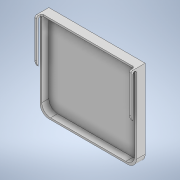
# Autodesk Inventor part: backpack
Saved by Autodesk Inventor 2021 (Build 250183000, 183)
## iProperties
Created: 2021-02-06
Part Number: backpack
Material: Generic
Document SubType Name: Modeling
Designer: allen
Density: 1 g/cm^3
Appearance: Default
Author: allen
Autodesk Inventor part; units mm, degrees
ref_plane "YZ Plane" through (0, 0, 0) normal (1, 0, 0) x (0, 1, 0)
ref_plane "XZ Plane" through (0, 0, 0) normal (0, 1, 0) x (-1, 0, 0)
ref_plane "XY Plane" through (0, 0, 0) normal (0, 0, 1) x (1, 0, 0)
sketch "Sketch1" plane through (0, 0, 0) normal (0, 0, 1) x (1, 0, 0)
  line L0 (55, -50) -> (-55, -50)
  line L1 (-55, -50) -> (-55, 50)
  line L2 (-55, 50) -> (55, 50)
  line L3 (55, 50) -> (55, -50)
  line L4 (55, -50) -> (-55, 50) construction
  line L5 (-55, -50) -> (55, 50) construction
  point P0 (0, 0)
  dimension "d0" = 110
  dimension "d1" = 100
  constraints: 12 end point, 2 midpoint, 2 parallel, 1 horizontal, 1 perpendicular
  measures "d0" distance of L1.end L2.end
  measures "d1" distance of L0.end L1.end
extrude "Extrusion1" add sketch "Sketch1" along normal blind 10
sketch "Sketch2" plane through (0, 0, 10) normal (0, 0, 1) x (1, 0, 0)
  line L0 (53, -48) -> (-53, -48)
  line L1 (-53, -48) -> (-53, 48)
  line L2 (-53, 48) -> (53, 48)
  line L3 (53, 48) -> (53, -48)
  line L4 (53, -48) -> (-53, 48) construction
  line L5 (-53, -48) -> (53, 48) construction
  point P0 (0, 0)
  dimension "d4" = 106
  dimension "d5" = 96
  constraints: 12 end point, 2 midpoint, 2 parallel, 1 horizontal, 1 perpendicular
  measures "d4" distance of L1.end L2.end
  measures "d5" distance of L0.end L1.end
extrude "Extrusion2" cut sketch "Sketch2" against normal blind 8
fillet "Fillet1" radius 10 4 edges at (-55, -50, 5) (-53, -48, 6) (55, -50, 5) (53, -48, 6)
sketch "Sketch3" plane through (-55, 50, 0) normal (-1, 0, 0) x (0, 0, 1)
  line L0 (0, 0) -> (10, 0) projected
  line L1 (10, 0) -> (16, 0)
  line L2 (16, 0) -> (16, -50)
  line L3 (16, -50) -> (14, -50)
  line L4 (14, -50) -> (14, -2)
  line L5 (14, -2) -> (10, -2)
  line L6 (10, -90) -> (10, 0) projected
  point P0 (0, -50)
  dimension "d9" = 50
  dimension "d10" = 6
  dimension "d11" = 4
  dimension "d12" = 2
  constraints: 10 end point, 3 perpendicular, 1 horizontal, 1 parallel, 1 point on line
  measures "d9" distance of L1.end L2.end
  measures "d10" distance of L0.end L1.end
  measures "d11" distance of L4.end L5.end
  measures "d12" distance between parallel lines of L1 L5
extrude "Extrusion3" add sketch "Sketch3" against normal blind 2
sketch "Sketch4" plane through (55, 50, 10) normal (1, 0, 0) x (0, 0, -1)
  line L0 (10, 0) -> (0, 0) projected
  line L1 (10, 0) -> (-6, 0) projected
  line L2 (0, 0) -> (-6, 0)
  line L3 (-6, 0) -> (-6, -50) projected
  line L4 (-6, 0) -> (-6, -50)
  line L5 (-6, -50) -> (-4, -50) projected
  line L6 (-6, -50) -> (-4, -50)
  line L7 (-4, -50) -> (-4, -2) projected
  line L8 (-4, -50) -> (-4, -2)
  line L9 (-4, -2) -> (0, -2)
  line L10 (0, -90) -> (0, 0) projected
  point P0 (10, -50)
  constraints: 10 end point, 3 perpendicular, 1 collinear, 1 horizontal, 1 point on line
extrude "Extrusion4" add sketch "Sketch4" against normal blind 2
fillet "Fillet2" radius 10 2 edges at (-54, 0, 16) (54, 0, 16)
fillet "Fillet3" radius 2 8 edges at (-54, 50, 16) (54, 50, 16) (-54, 48, 14) (54, 48, 14) (54, 48, 10) (-54, 48, 10) (-53, 49, 10) (53, 49, 10)
body "Solid1"
